Autodesk Inventor part; units mm, degrees
(part 2 of 2)
extrude "Extrusion12" cut sketch "Sketch6" against normal through all contours L210 A2 L206 L1 L0 A0 | A0 L0 L1 L206 L103 A30 L210 | A30 L103 L100 L101 L129 L208 L209 L210 | L210 A2 L206 | L210 A31 L107 L206 L5 L6 A1 | A1 L6 L5 L206 A2 L210 | A30 L131 L130 L129 L101 L100 L103 | L103 L102 L101 L129 L130 L131 A30 | L206 A2 | A2 L206 L5 L4 L204 L2 L1 | L210 L134 L107 A31 | L1 L2 L204 L102 L206 | A31 L125 L126 L127 L105 L104 L107 | L107 L134 L133 L132 A32 L105 L127 L126 L125 A31 | L210 L136 L99 L206 L10 L11 L12 L107 L134 | L204 L2 L3 L4 L105 L127 L208 L129 L101 | L206 L104 L204 L4 L5 | L107 L106 L105 A32 L132 L133 L134 | L210 A34 L99 L136 | L204 L4 L3 L2 | L127 L105 A32 L208 | L206 L12 L13 L204 L106 | L136 L137 L138 A33 L97 L96 L99 | L99 A34 L147 L146 L145 L97 A33 L138 L137 L136 | L210 A6 L16 L17 L206 L99 A34 | A32 L105 L204 L13 L14 A4 L208 | L206 L10 L9 L204 A5 L13 L12 | L12 L11 L10 L206 | L96 L204 L9 L10 L206 | L99 L98 L97 L145 L146 L147 A34 | L210 A8 L206 L17 L16 A6 | A4 L14 L13 L204 A5 L208 | L97 A33 L208 A3 L8 L9 L204 | L206 L17 L18 L204 L98 | L210 A8 L206 | A5 L204 L208 | A5 L204 | L97 L145 L208 A33 | L9 L8 A3 L208 A5 L204 | L204 L18 L19 L20 L113 L143 L208 L145 L97 | L206 A8 L21 L20 L204 L18 L17 | L210 L150 L115 A35 | A35 L115 L206 L21 L22 A7 L210 | L210 A7 L22 L21 L206 A8 | L206 A8 | L204 L20 L19 L18 | A35 L141 L142 L143 L113 L112 L115 | L115 L150 L149 L148 A36 L113 L143 L142 L141 A35 | L210 L152 L111 L206 L26 L27 L28 L115 L150 | L20 L21 L206 L112 L204 | L115 L114 L113 A36 L148 L149 L150 | L210 A39 L111 L152 | L143 L113 A36 L208 | L206 L28 L29 L204 L114 | L152 L153 L154 A37 L109 L108 L111 | L111 A39 L162 L161 L160 L109 A37 L154 L153 L152 | L210 A12 L32 L33 L206 L111 A39 | A36 L113 L204 L29 L30 A10 L208 | L206 L26 L25 L204 A11 L29 L28 | L28 L27 L26 L206 | L108 L204 L25 L26 L206 | L111 L110 L109 L160 L161 L162 A39 | L210 A14 L206 L33 L32 A12 | A10 L30 L29 L204 A11 L208 | L109 A37 L208 A9 L24 L25 L204 | L206 L33 L34 L204 L110 | L210 A14 L206 | A11 L204 L208 | A11 L204 | L109 L160 L208 A37 | L25 L24 A9 L208 A11 L204 | L204 L34 L35 L36 L81 L158 L208 L160 L109 | L206 A14 L37 L36 L204 L34 L33 | L210 L166 L83 A38 | A38 L83 L206 L37 L38 A13 L210 | L210 A13 L38 L37 L206 A14 | L206 A14 | L204 L36 L35 L34 | A38 L156 L157 L158 L81 L80 L83 | L83 L166 L165 L164 A40 L81 L158 L157 L156 A38 | L210 L168 L87 L206 L42 L43 L44 L83 L166 | L36 L37 L206 L80 L204 | L83 L82 L81 A40 L164 L165 L166 | L210 A42 L87 L168 | L158 L81 A40 L208 | L206 L44 L45 L204 L82 | L168 L169 L170 A41 L85 L84 L87 | L87 A42 L179 L178 L177 L85 A41 L170 L169 L168 | L210 A18 L48 L49 L206 L87 A42 | A40 L81 L204 L45 L46 A16 L208 | L206 L42 L41 L204 A17 L45 L44 | L44 L43 L42 L206 | L84 L204 L41 L42 L206 | L87 L86 L85 L177 L178 L179 A42 | L210 A20 L206 L49 L48 A18 | A16 L46 L45 L204 A17 L208 | L85 A41 L208 A15 L40 L41 L204 | L206 L49 L50 L204 L86 | L210 A20 L206 | A17 L204 L208 | A17 L204 | L85 L177 L208 A41 | L41 L40 A15 L208 A17 L204 | L204 L50 L51 L52 L121 L175 L208 L177 L85 | L206 A20 L53 L52 L204 L50 L49 | L210 L182 L123 A43 | A43 L123 L206 L53 L54 A19 L210 | L210 A19 L54 L53 L206 A20 | L206 A20 | L204 L52 L51 L50 | A43 L173 L174 L175 L121 L120 L123 | L123 L182 L181 L180 A44 L121 L175 L174 L173 A43 | L210 L184 L91 L206 L58 L59 L60 L123 L182 | L52 L53 L206 L120 L204 | L123 L122 L121 A44 L180 L181 L182 | L210 A46 L91 L184 | L175 L121 A44 L208 | L206 L60 L61 L204 L122 | L184 L185 L186 A45 L89 L88 L91 | L91 A46 L195 L194 L193 L89 A45 L186 L185 L184 | L210 A24 L64 L65 L206 L91 A46 | A44 L121 L204 L61 L62 A22 L208 | L206 L58 L57 L204 A23 L61 L60 | L60 L59 L58 L206 | L88 L204 L57 L58 L206 | L91 L90 L89 L193 L194 L195 A46 | L210 A26 L206 L65 L64 A24 | A22 L62 L61 L204 A23 L208 | L89 A45 L208 A21 L56 L57 L204 | L206 L65 L66 L204 L90 | L210 A26 L206 | A23 L204 L208 | A23 L204 | L89 L193 L208 A45 | L57 L56 A21 L208 A23 L204 | L204 L66 L67 L68 L117 L191 L208 L193 L89 | L206 A26 L69 L68 L204 L66 L65 | L210 L198 L119 A47 | A47 L119 L206 L69 L70 A25 L210 | L210 A25 L70 L69 L206 A26 | L206 A26 | L204 L68 L67 L66 | A47 L189 L190 L191 L117 L116 L119 | L119 L198 L197 L196 A48 L117 L191 L190 L189 A47 | L210 L200 L95 L206 L74 L75 L76 L119 L198 | L68 L69 L206 L116 L204 | L119 L118 L117 A48 L196 L197 L198 | L210 L211 L208 A49 L93 L94 L95 L200 | L191 L117 A48 L208 | L206 L76 L77 L204 L118 | L200 L201 L202 A49 L93 L92 L95 | L95 L94 L93 A49 L202 L201 L200 | A48 L117 L204 L77 L78 A28 L208 | L206 L74 L73 L204 A29 L77 L76 | L76 L75 L74 L206 | L92 L204 L73 L74 L206 | A28 L78 L77 L204 A29 L208 | L93 A49 L208 A27 L72 L73 L204 | A29 L204 L208 | A29 L204 | L73 L72 A27 L208 A29 L204
extrude "Extrusion13" cut sketch "Sketch8" against normal through all contours L134 A2 L120 L1 L0 A0 | A0 L0 L1 L120 L103 A40 L134 | A40 L103 L165 L134 | L134 A2 L120 | L134 A41 L107 L120 L5 L6 A1 | A1 L6 L5 L120 A2 L134 | L165 L103 L120 L10 L11 L12 L163 L134 | A40 L175 L174 L173 L101 A38 L167 L166 L165 L103 | L103 L102 L101 L173 L174 L175 A40 | L120 A2 | A2 L120 L5 L4 L122 L2 L1 | L134 L179 L107 A41 | L1 L2 L122 L102 L120 | L163 L120 A37 L134 | L165 L166 L167 A38 L101 L100 L103 | L134 L181 L111 L120 L74 L75 L76 L107 L179 | A41 L169 L170 L171 L105 L104 L107 | L107 L179 L178 L177 A43 L105 L171 L170 L169 A41 | A37 L120 L21 L22 A7 L134 | L163 L162 L161 A39 L122 L155 L154 L153 A37 L120 | L120 L12 L13 L122 A39 L161 L162 L163 | L100 L122 L9 L10 L120 | L122 L2 L3 L4 L105 L171 L132 L173 L101 | L120 L104 L122 L4 L5 | L134 A44 L111 L181 | L107 L106 L105 A43 L177 L178 L179 | L122 L4 L3 L2 | A7 L22 L21 L120 A8 L134 | A37 L153 L154 L155 L122 L20 L21 L120 | L120 L10 L9 L122 A5 L13 L12 | L12 L11 L10 L120 | L101 A38 L132 A3 L8 L9 L122 | L173 L132 A38 L101 | L134 A24 L64 L65 L120 L111 A44 | L181 L182 L183 A42 L109 L108 L111 | L111 A44 L191 L190 L189 L109 A42 L183 L182 L181 | L120 L76 L77 L122 L106 | A8 L120 L134 | L21 L20 L122 L18 L17 L120 A8 | L9 L8 A3 L132 A5 L122 | L134 A26 L120 L65 L64 A24 | L111 L110 L109 L189 L190 L191 A44 | L108 L122 L73 L74 L120 | L122 L77 L78 A28 L132 A43 L105 | L120 L74 L73 L122 A29 L77 L76 | L76 L75 L74 L120 | L105 A43 L132 L171 | A8 L120 L17 L16 A6 L134 | A8 L120 | A36 L99 L149 L134 | L134 A6 L16 L17 L120 L99 A36 | L122 A5 L132 A4 L14 L13 | L13 L14 A4 L132 A39 L122 | L122 A5 | A5 L132 L122 | L134 A26 L120 | L120 L65 L66 L122 L110 | L109 A42 L132 A27 L72 L73 L122 | L122 A29 L132 A28 L78 L77 | L122 L155 L132 L157 L97 L18 L19 L20 | L20 L19 L18 L122 | L149 L99 L120 L26 L27 L28 L95 L147 L134 | A36 L159 L158 L157 L97 A34 L151 L150 L149 L99 | L99 L98 L97 L157 L158 L159 A36 | A39 L132 L155 L122 | L134 A25 L70 L69 L120 A26 | L120 A26 | A26 L120 L69 L68 L122 L66 L65 | A45 L119 L120 L69 L70 A25 L134 | L134 L195 L119 A45 | L122 L66 L67 L68 L117 L187 L132 L189 L109 | L109 L189 L132 A42 | L73 L72 A27 L132 A29 L122 | L122 A29 L132 | A29 L122 | L17 L18 L122 L98 L120 | L147 L95 A33 L134 | L149 L150 L151 A34 L97 L96 L99 | L134 L197 L115 L120 L58 L59 L60 L119 L195 | A45 L185 L186 L187 L117 L116 L119 | L119 L195 L194 L193 A47 L117 L187 L186 L185 A45 | L122 L68 L67 L66 | A33 L95 L120 L37 L38 A13 L134 | L147 L146 L145 A35 L93 L139 L138 L137 A33 L95 | L95 L94 L93 A35 L145 L146 L147 | L96 L122 L25 L26 L120 | L120 L116 L122 L68 L69 | L134 A48 L115 L197 | L119 L118 L117 A47 L193 L194 L195 | L157 L132 A34 L97 | A13 L38 L37 L120 A14 L134 | A33 L137 L138 L139 L93 L92 L95 | L120 L28 L29 L122 L94 | L97 A34 L132 A9 L24 L25 L122 | L120 L28 L27 L26 | L26 L25 L122 A11 L29 L28 L120 | L134 A18 L48 L49 L120 L115 A48 | L197 L198 L199 A46 L113 L112 L115 | L115 A48 L207 L206 L205 L113 A46 L199 L198 L197 | L120 L60 L61 L122 L118 | L187 L117 A47 L132 | A14 L120 L134 | L92 L122 L36 L37 L120 | L122 L29 L30 A10 L132 A35 L93 | L25 L24 A9 L132 A11 L122 | L134 A20 L120 L49 L48 A18 | L115 L114 L113 L205 L206 L207 A48 | L112 L122 L57 L58 L120 | L122 L61 L62 A22 L132 A47 L117 | L120 L58 L57 L122 A23 L61 L60 | L60 L59 L58 L120 | A14 L120 L33 L32 A12 L134 | L120 L37 L36 L122 L34 L33 A14 | A14 L120 | L93 L139 L132 L141 L89 L122 L34 L35 L36 | A32 L91 L128 L134 | L134 A12 L32 L33 L120 L91 A32 | A35 L132 L139 L93 | L122 A11 L132 A10 L30 L29 | L122 A11 | A11 L132 L122 | L134 A20 L120 | L120 L49 L50 L122 L114 | L113 A46 L132 A21 L56 L57 L122 | L122 A23 L132 A22 L62 L61 | L36 L35 L34 L122 | L128 L91 L120 L42 L43 L44 L87 L126 L134 | A32 L143 L142 L141 L89 A31 L130 L129 L128 L91 | L91 L90 L89 L141 L142 L143 A32 | L134 A19 L54 L53 L120 A20 | L120 A20 | A20 L120 L53 L52 L122 L50 L49 | A49 L83 L120 L53 L54 A19 L134 | L134 L135 L132 L203 L81 L82 L83 A49 | L122 L50 L51 L52 L81 L203 L132 L205 L113 | L113 L205 L132 A46 | L57 L56 A21 L132 A23 L122 | L122 A23 L132 | A23 L122 | L33 L34 L122 L90 L120 | L128 L129 L130 A31 L89 L88 L91 | L126 L87 L84 L85 A30 L132 L133 L134 | A49 L201 L202 L203 L81 L80 L83 | L83 L82 L81 L203 L202 L201 A49 | L122 L52 L51 L50 | L132 A31 L89 L141 | L88 L122 L41 L42 L120 | L126 L125 L124 A30 L85 L84 L87 | L87 L86 L85 A30 L124 L125 L126 | L120 L80 L122 L52 L53 | L132 A15 L40 L41 L122 L89 A31 | L120 L44 L43 L42 | L42 L41 L122 A17 L45 L44 L120 | L120 L44 L45 L122 L86 | L132 A17 L122 L41 L40 A15 | L122 L45 L46 A16 L132 A30 L85 | L132 A17 L122 | L122 A17 | L122 A17 L132 A16 L46 L45
sketch "Sketch27" plane through (31.8897, 11.2835, -25.977) normal (0, 0, -1) x (-1, 0, 0)
  line L0 (58.9982, -8.9716) -> (8.6847, -8.9716) projected
  line L1 (8.6847, -8.9716) -> (8.6847, -6.9702) projected
  line L2 (8.6847, -6.9702) -> (58.9982, -6.9702) projected
  line L3 (58.9982, -6.9702) -> (58.9982, -8.9716) projected
  line L4 (4.7812, -15.6059) -> (4.7812, -13.6045) projected
  line L5 (4.7812, -13.6045) -> (55.0947, -13.6045) projected
  line L6 (55.0947, -13.6045) -> (55.0947, -15.6059) projected
  line L7 (55.0947, -15.6059) -> (4.7812, -15.6059) projected
  arc A0 (63.7794, -22.567) -> (68.9542, -17.3922) centre (63.7794, -17.3922) ccw projected
  line L8 (68.9542, -5.1748) -> (68.9542, -17.3922) projected
  arc A1 (68.9542, -5.1748) -> (63.7794, 0) centre (63.7794, -5.1748) ccw projected
  line L9 (0, 0) -> (63.7794, 0) projected
  arc A2 (0, 0) -> (-5.1748, -5.1748) centre (0, -5.1748) ccw projected
  line L10 (-5.1748, -17.3922) -> (-5.1748, -5.1748) projected
  arc A3 (-5.1748, -17.3922) -> (0, -22.567) centre (0, -17.3922) ccw projected
  line L11 (63.7794, -22.567) -> (0, -22.567) projected
  point P0 (31.8897, -11.2835)
extrude "Extrusion14" cut sketch "Sketch27" against normal blind 7.62 contours L0 L1 L2 L3 | L4 L5 L6 L7 | L11 A3 L10 A2 L9 A1 L8 A0
sketch "Sketch29" plane through (-21.3801, -2.5043, -26.2897) normal (0, -0.0871557, -0.9961947) x (1, 0, 0)
  line L0 (45.4885, -1.4254) -> (1.175, -1.4254)
  line L1 (1.175, -1.4254) -> (1.175, 3.1084)
  line L2 (1.175, 3.1084) -> (45.4885, 3.1084)
  line L3 (45.4885, 3.1084) -> (45.4885, -1.4254)
  line L4 (48.4885, -0.1554) -> (48.4885, 1.8384) projected
  line L5 (-1.825, 1.8384) -> (-1.825, -0.1554) projected
  line L6 (48.4885, 1.8384) -> (-1.825, 1.8384) projected
  line L7 (-1.825, -0.1554) -> (48.4885, -0.1554) projected
  point P0 (21.3801, -0.2035)
  dimension "d150" = 3
  dimension "d151" = 3
  dimension "d152" = 1.27
  dimension "d153" = 1.27
  constraints: 8 end point, 2 parallel, 1 horizontal, 1 perpendicular
  measures "d150" distance between parallel lines of L3 L4
  measures "d151" distance between parallel lines of L5 L1
  measures "d152" distance between parallel lines of L6 L2
  measures "d153" distance between parallel lines of L7 L0
extrude "Extrusion15" cut sketch "Sketch29" against normal through all contours L0 L1 L7 L3 | L7 L1 L6 L3 | L6 L1 L2 L3
sketch "Sketch30" plane through (22.2277, 2.6133, -26.3842) normal (0, 0.0871557, -0.9961947) x (-1, 0, 0)
  line L0 (2.0226, 2.999) -> (46.3361, 2.999)
  line L1 (46.3361, 2.999) -> (46.3361, -1.5348)
  line L2 (46.3361, -1.5348) -> (2.0226, -1.5348)
  line L3 (2.0226, -1.5348) -> (2.0226, 2.999)
  line L4 (-0.9774, 1.729) -> (-0.9774, -0.2648) projected
  line L5 (49.3361, -0.2648) -> (49.3361, 1.729) projected
  line L6 (49.3361, 1.729) -> (-0.9774, 1.729) projected
  line L7 (-0.9774, -0.2648) -> (49.3361, -0.2648) projected
  point P0 (22.2277, -0.3039)
  dimension "d156" = 3
  dimension "d157" = 3
  dimension "d158" = 1.27
  dimension "d159" = 1.27
  constraints: 8 end point, 2 parallel, 1 horizontal, 1 perpendicular
  measures "d156" distance between parallel lines of L4 L3
  measures "d157" distance between parallel lines of L5 L1
  measures "d158" distance between parallel lines of L0 L6
  measures "d159" distance between parallel lines of L7 L2
extrude "Extrusion16" cut sketch "Sketch30" against normal through all contours L0 L1 L6 L3 | L6 L1 L7 L3 | L7 L1 L2 L3
sketch "Sketch31" plane through (31.8897, 11.2835, -18.357) normal (0, 0, -1) x (-1, 0, 0)
  line L0 (55.9982, -10.9131) -> (11.6847, -10.9131) projected
  line L1 (7.7812, -11.663) -> (52.0947, -11.663) projected
  line L2 (-20.0006, -11.2835) -> (83.78, -11.2835) projected
  line L3 (7.7812, -12.9378) -> (7.7812, -11.663) projected
  line L4 (7.7812, -11.663) -> (7.7812, -11.2835)
  line L5 (11.6847, -10.9131) -> (11.6847, -11.2835)
  line L6 (55.9982, -10.9131) -> (55.9982, -11.109)
  line L7 (55.9982, -11.7465) -> (55.9982, -10.4716) projected
  line L8 (52.0947, -11.663) -> (52.0947, -11.2835)
  point P0 (31.8897, -11.2835)
  point P1 (55.9982, -11.2835)
  constraints: 8 end point, 3 point on line, 2 perpendicular, 1 collinear, 1 midpoint
extrude "Extrusion17" cut sketch "Sketch31" against normal through all
sketch "Sketch32" plane through (31.8897, 11.2835, -18.357) normal (0, 0, -1) x (-1, 0, 0)
  line L0 (0, 0) -> (63.7794, 0) projected
  line L1 (63.7794, -22.567) -> (0, -22.567) projected
  line L2 (-5.1748, -17.3922) -> (-5.1748, -5.1748) projected
  line L3 (68.9542, -5.1748) -> (68.9542, -17.3922) projected
  arc A0 (0, 0) -> (-5.1748, -5.1748) centre (0, -5.1748) ccw projected
  line L4 (0, 0) -> (-5.1748, 0)
  line L5 (-5.1748, 0) -> (-5.1748, -5.1748)
  line L6 (-5.1748, -5.1748) -> (-5.1748, -22.567)
  arc A1 (-5.1748, -17.3922) -> (0, -22.567) centre (0, -17.3922) ccw projected
  line L7 (-5.1748, -22.567) -> (0, -22.567)
  line L8 (0, -22.567) -> (68.9542, -22.567)
  arc A2 (63.7794, -22.567) -> (68.9542, -17.3922) centre (63.7794, -17.3922) ccw projected
  line L9 (68.9542, -22.567) -> (68.9542, -17.3922)
  line L10 (68.9542, -17.3922) -> (68.9542, 0)
  arc A3 (68.9542, -5.1748) -> (63.7794, 0) centre (63.7794, -5.1748) ccw projected
  line L11 (63.7794, 0) -> (68.9542, 0)
  point P0 (31.8897, -11.2835)
  constraints: 16 end point, 7 tangent, 4 perpendicular, 4 point on line, 1 horizontal
extrude "Extrusion18" add sketch "Sketch32" against normal up to surface (19.557 mm away) contours A0 L5 L4 | L11 L10 A3 | A1 L7 L6 | L9 L8 A2
sketch "Sketch33" plane through (37.0645, -11.2835, 1.2) normal (1, 0, 0) x (0, 0, -1)
  line L0 (19.557, 22.567) -> (0, 22.567) projected
  line L1 (19.557, 0) -> (0, 0) projected
  line L2 (2.8, 3.8924) -> (10.032, 3.8924) projected
  line L3 (2.8, 18.6747) -> (10.032, 18.6747) projected
  line L4 (10.032, 15.3717) -> (10.032, 14.0968) projected
  line L5 (10.032, 14.0968) -> (10.032, 12.0954) projected
  line L6 (10.032, 12.0954) -> (10.032, 11.7373) projected
  line L7 (10.032, 11.7373) -> (10.032, 10.4625) projected
  line L8 (10.032, 10.4625) -> (10.032, 8.4611) projected
  line L9 (10.032, 8.4611) -> (10.032, 7.1862) projected
  line L10 (10.032, 7.1862) -> (10.032, 8.4611) projected
  line L11 (10.032, 8.4611) -> (10.032, 10.4625) projected
  line L12 (10.032, 10.4625) -> (10.032, 10.8205) projected
  line L13 (10.032, 10.8205) -> (10.032, 12.0954) projected
  line L14 (10.032, 12.0954) -> (10.032, 14.0968) projected
  line L15 (10.032, 14.0968) -> (10.032, 15.3717) projected
  line L16 (10.032, 11.2835) -> (10.032, 8.2968) projected
  line L17 (10.032, 18.6747) -> (10.032, 11.2835) projected
  line L18 (10.032, 18.6747) -> (10.032, 18.6747) projected
  line L19 (10.032, 14.2702) -> (10.032, 18.6747) projected
  line L20 (10.032, 11.2835) -> (10.032, 14.2702) projected
  line L21 (10.032, 8.2968) -> (10.032, 11.2835) projected
  line L22 (10.032, 3.8924) -> (10.032, 8.2968) projected
  line L23 (10.032, 8.2968) -> (10.032, 3.8924) projected
  line L24 (19.557, 22.567) -> (19.557, 0) projected
  line L25 (10.032, 18.6747) -> (10.032, 18.6747) projected
  line L26 (19.557, 16.205) -> (10.032, 15.3717) projected
  line L27 (19.557, 16.205) -> (10.032, 15.3717) projected
  line L28 (10.032, 15.3717) -> (10.032, 14.0968) projected
  line L29 (10.032, 15.3717) -> (19.557, 22.567)
  point P0 (1.2, 11.2835)
  point P1 (14.7945, 18.9693)
  constraints: 2 end point, 1 midpoint, 1 other
hole "Hole11" at (37.0645, 7.6858, -13.5945) direction (-1, 0, 0) diameter 3.4036 depth 37.0586 tip angle 118 counterbore diameter 5.5 counterbore depth 30.7086 clearance for "Socket Head Cap Screw" size "M3" standard "Ansi Metric M Profile"
sketch "Sketch34" plane through (37.0645, -11.2835, 1.2) normal (1, 0, 0) x (0, 0, -1)
  circle A0 centre (14.7945, 18.9693) radius 1.7018 projected
  point P0 (1.2, 11.2835)
hole "Hole12" at (37.0645, 7.6858, -13.5945) direction (-1, 0, 0) diameter 2.459 end through all thread size "M3x0.5" class "6H" standard "ANSI Metric M Profile"
pattern_circular "Circular Pattern3" count 2 over 360 about axis through (0, 0, -10) along (0, 0, 1) of "Hole11", "Hole12"
split body "Split8" result two bodies by plane through (0, 0, 0) normal (1, 0, 0) first body at (12.3548, 10.7835, -5.319)
body "Solid16"
body "Solid17"
